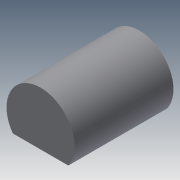
# Autodesk Inventor part: speaker_body
Saved by Autodesk Inventor 2015 (Build 190159000, 159)
## iProperties
Created: 2018-01-22
Part Number: speaker_body
Material: Generic
Document SubType Name: Modeling
Designer: rissa
Density: 1 g/cm^3
Appearance: Default
Author: rissa
Autodesk Inventor part; units mm, degrees
ref_plane "YZ Plane" through (0, 0, 0) normal (1, 0, 0) x (0, 1, 0)
ref_plane "XZ Plane" through (0, 0, 0) normal (0, 1, 0) x (-1, 0, 0)
ref_plane "XY Plane" through (0, 0, 0) normal (0, 0, 1) x (1, 0, 0)
sketch "Sketch1" plane through (0, 0, 0) normal (0, 0, 1) x (1, 0, 0)
  circle A0 centre (0, 0) radius 27.5
  dimension "d0" = 55
  constraints: 1 centre point, 1 coincident
  measures "d0" diameter of A0
extrude "Extrusion1" add sketch "Sketch1" along normal blind 80
sketch "Sketch2" plane through (0, 0, 80) normal (0, 0, 1) x (1, 0, 0)
  circle A0 centre (0, 0) radius 27.5 projected
  line L0 (-22.5, -15.8114) -> (22.5, -15.8114)
  dimension "d5" = 45
  constraints: 2 end point, 2 point on circle, 1 horizontal
  measures "d5" distance of L0.start L0.end
extrude "Extrusion2" cut sketch "Sketch2" against normal blind 80 contours L0 A0 picked at (-6.0353, -17.4405)
sketch "Sketch3" plane through (-22.5, -15.8114, 80) normal (0, -1, 0) x (1, 0, 0)
  line L0 (43, -70) -> (2, -70)
  line L1 (2, -70) -> (2, -29)
  line L2 (2, -29) -> (43, -29)
  line L3 (43, -29) -> (43, -70)
  line L4 (0, -80) -> (0, 0) projected
  line L5 (45, 0) -> (45, -80) projected
  line L6 (0, 0) -> (45, 0) projected
  line L7 (45, -80) -> (0, -80) projected
  point P0 (22.5, -80)
  dimension "d16" = 41
  dimension "d17" = 41
  dimension "d18" = 45
  dimension "d19" = 2
  dimension "d20" = 29
  constraints: 8 end point, 2 parallel, 1 horizontal, 1 perpendicular
  measures "d16" distance of L1.end L2.end
  measures "d17" distance between parallel lines of L2 L0
  measures "d18" distance between parallel lines of L4 L5
  measures "d19" distance between parallel lines of L4 L1
  measures "d20" distance between parallel lines of L6 L2
extrude "Extrusion3" cut sketch "Sketch3" against normal blind 1.5 contours L0 L1 L2 L3
sketch "Sketch4" plane through (0, 0, 0) normal (0, 0, -1) x (-1, 0, 0)
  arc A0 (22.5, -15.8114) -> (-22.5, -15.8114) centre (0, 0) ccw projected
  circle A1 centre (0, 0) radius 25
  line L0 (21.4678, -12.8114) -> (-21.4678, -12.8114)
  line L1 (-22.5, -15.8114) -> (22.5, -15.8114) projected
  dimension "d12" = 50
  dimension "d13" = 3
  constraints: 2 end point, 2 point on circle, 1 centre point, 1 coincident, 1 horizontal
  measures "d12" diameter of A1
  measures "d13" distance between parallel lines of L0 L1
extrude "Extrusion4" cut sketch "Sketch4" against normal blind 77 contours L0 A1
sketch "Sketch5" plane through (-22.5, -14.3114, 80) normal (0, -1, 0) x (1, 0, 0)
  circle A0 centre (22.5, -50.1203) radius 18
  point P0 (22.5, -80)
  dimension "d25" = 36
  constraints: 1 centre point
  measures "d25" diameter of A0
extrude "Extrusion5" cut sketch "Sketch5" against normal blind 31
hole "Hole1" at (-17.5, -14.3114, 48) direction (0, 1, 0) diameter 3 depth 8
hole "Hole2" at (17.5, -14.3114, 48) direction (0, 1, 0) diameter 3 depth 8
hole "Hole3" at (-17.5, -14.3114, 13) direction (0, 1, 0) diameter 3 depth 8
hole "Hole4" at (17.5, -14.3114, 13) direction (0, 1, 0) diameter 3 depth 8
body "Solid1"
